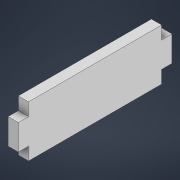
# Autodesk Inventor part: Кусочек барабана
Saved by Autodesk Inventor 2022 (Build 260153000, 153)
## iProperties
Created: 2023-02-11
Part Number: Кусочек барабана
Material: Типовые
Document SubType Name: Modeling
Designer: Глеб
Density: 1 g/cm^3
Appearance: По умолчанию
Author: Глеб
Autodesk Inventor part; units mm, degrees
ref_plane "YZ Plane" through (0, 0, 0) normal (1, 0, 0) x (0, 1, 0)
ref_plane "XZ Plane" through (0, 0, 0) normal (0, 1, 0) x (-1, 0, 0)
ref_plane "XY Plane" through (0, 0, 0) normal (0, 0, 1) x (1, 0, 0)
sketch "Эскиз1" plane through (0, 0, 0) normal (1, 0, 0) x (0, 1, 0)
  line L0 (0, -42) -> (0, 42) construction
  line L1 (-10, -26) -> (10, -26)
  line L2 (10, -26) -> (10, 26)
  line L3 (10, 26) -> (-10, 26)
  line L4 (-10, 26) -> (-10, -26)
  line L5 (-10, -26) -> (10, 26) construction
  line L6 (10, -26) -> (-10, 26) construction
  line L7 (5, 30) -> (-5, 30)
  line L8 (-5, 30) -> (-5, 26)
  line L9 (-5, 26) -> (5, 26)
  line L10 (5, 26) -> (5, 30)
  line L11 (5, -26) -> (-5, -26)
  line L12 (-5, -26) -> (-5, -30)
  line L13 (-5, -30) -> (5, -30)
  line L14 (5, -30) -> (5, -26)
  point P0 (0, 0)
  dimension "d3" = 20
  dimension "d4" = 60
  dimension "d5" = 4
  dimension "d6" = 10
  constraints: 28 end point, 6 parallel, 3 collinear, 3 horizontal, 3 perpendicular, 2 midpoint, 2 point on line, 1 other
  measures "d3" distance of L1.start L1.end
  measures "d4" distance between parallel lines of L13 L7
  measures "d5" distance between parallel lines of L13 L1
  measures "d6" distance of L12.end L13.end
extrude "Выдавливание1" add sketch "Эскиз1" along normal mid plane 4
